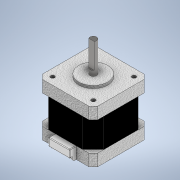
# Autodesk Inventor part: Шаговый двигатель
Saved by Autodesk Inventor 2020 (Build 240168000, 168)
## iProperties
Created: 2020-12-07
Part Number: Шаговый двигатель
Material: Типовые
Document SubType Name: Modeling
Designer: User
Density: 1 g/cm^3
Appearance: По умолчанию
Author: User
Autodesk Inventor part; units mm, degrees
ref_plane "YZ Plane" through (0, 0, 0) normal (1, 0, 0) x (0, 1, 0)
sketch "Эскиз1" plane through (0, 0, 0) normal (0, 1, 0) x (-1, 0, 0)
  line L0 (21.1, 21.1) -> (-21.1, 21.1)
  line L1 (-21.1, 21.1) -> (-21.1, -21.1)
  line L2 (-21.1, -21.1) -> (21.1, -21.1)
  line L3 (21.1, -21.1) -> (21.1, 21.1)
  line L4 (21.1, 21.1) -> (-21.1, -21.1) construction
  line L5 (-21.1, 21.1) -> (21.1, -21.1) construction
  line L6 (-15.5, -15.5) -> (15.5, -15.5) construction
  line L7 (15.5, -15.5) -> (15.5, 15.5) construction
  line L8 (15.5, 15.5) -> (-15.5, 15.5) construction
  line L9 (-15.5, 15.5) -> (-15.5, -15.5) construction
  line L10 (-15.5, -15.5) -> (15.5, 15.5) construction
  line L11 (15.5, -15.5) -> (-15.5, 15.5) construction
  circle A0 centre (15.5, -15.5) radius 1.5
  circle A1 centre (-15.5, -15.5) radius 1.5
  circle A2 centre (15.5, 15.5) radius 1.5
  circle A3 centre (-15.5, 15.5) radius 1.5
  line L12 (21.1, 0) -> (-21.1, 0) construction
  line L13 (0, -21.1) -> (0, 21.1) construction
  point P0 (0, 0)
  dimension "d0" = 42.2
  dimension "d1" = 42.2
  dimension "d2" = 31
  dimension "d3" = 3
  constraints: 28 end point, 8 midpoint, 4 centre point, 4 coincident, 4 parallel, 3 equal radius, 3 perpendicular, 2 horizontal
  measures "d0" distance of L2.end L1.end
  measures "d1" distance of L1.end L0.end
  measures "d2" distance of L8.end L6.start
  measures "d3" diameter of A0
extrude "Выдавливание1" add sketch "Эскиз1" along normal blind 40
sketch "Эскиз2" plane through (0, 40, 0) normal (0, 1, 0) x (1, 0, 0)
  circle A0 centre (0, 0) radius 11
  dimension "d9" = 22
  constraints: 1 centre point, 1 coincident
  measures "d9" diameter of A0
extrude "Выдавливание2" add sketch "Эскиз2" along normal blind 2
sketch "Эскиз3" plane through (0, 42, 0) normal (0, 1, 0) x (1, 0, 0)
  circle A0 centre (0, 0) radius 2.5
  dimension "d12" = 5
  constraints: 1 centre point, 1 coincident
  measures "d12" diameter of A0
extrude "Выдавливание3" add sketch "Эскиз3" along normal blind 23
sketch "Эскиз4" plane through (0, 65, 0) normal (0, 1, 0) x (1, 0, 0)
  circle A0 centre (0, 0) radius 2.5 projected
  line L0 (-2.0766, -1.392) -> (2.0766, -1.392)
  line L1 (-2.4977, 0.108) -> (2.4977, 0.108) construction
  dimension "d15" = 1.5
  constraints: 4 end point, 4 point on circle, 2 horizontal
  measures "d15" distance between parallel lines of L0 L1
extrude "Выдавливание4" cut sketch "Эскиз4" against normal blind 19 contours L0 A0 picked at (0, -1.7613)
ref_plane "РабПлоскость1" through (0, 9, 0) normal (0, -1, 0) x (1, 0, 0)
ref_plane "РабПлоскость2" through (0, 31, 0) normal (0, 1, 0) x (1, 0, 0)
split body "Разделение1" result two bodies by plane through (0, 9, 0) normal (0, -1, 0) first body at (-4.7924, 0.5, 4.8351)
split body "Разделение2" result two bodies by plane through (0, 31, 0) normal (0, 1, 0) bodies 3 first body at (-4.7924, 31.5, -4.8351)
chamfer "Фаска1" distance 3.5 angle 45 8 edges at (-21.1, 4.5, 21.1) (-21.1, 4.5, -21.1) (21.1, 4.5, 21.1) (21.1, 4.5, -21.1) (-21.1, 35.5, -21.1) (-21.1, 35.5, 21.1) (21.1, 35.5, 21.1) (21.1, 35.5, -21.1)
chamfer "Фаска2" distance 8 angle 45 4 edges at (21.1, 20, -21.1) (-21.1, 20, -21.1) (21.1, 20, 21.1) (-21.1, 20, 21.1)
sketch "Эскиз5" plane through (-17.6, 0, 21.1) normal (0, 0, 1) x (1, 0, 0)
  line L0 (25.7, 0) -> (9.5, 0)
  line L1 (9.5, 0) -> (9.5, 9)
  line L2 (9.5, 9) -> (25.7, 9)
  line L3 (25.7, 9) -> (25.7, 0)
  line L4 (0, 0) -> (35.2, 0) projected
  line L5 (0, 9) -> (35.2, 9) projected
  point P0 (17.6, 0)
  point P1 (17.6, 0)
  dimension "d26" = 16.2
  constraints: 8 end point, 2 midpoint, 2 parallel, 1 collinear, 1 horizontal, 1 perpendicular
  measures "d26" distance of L1.end L2.end
extrude "Выдавливание5" add sketch "Эскиз5" along normal blind 5 separate body
sketch "Эскиз6" plane through (-17.6, 0, 26.1) normal (0, 0, 1) x (1, 0, 0)
  line L0 (9.5, 0) -> (25.7, 0)
  line L1 (25.7, 0) -> (25.7, 3)
  line L2 (25.7, 3) -> (9.5, 3)
  line L3 (9.5, 3) -> (9.5, 0)
  line L4 (9.5, 9) -> (9.5, 0) projected
  line L5 (0, 0) -> (35.2, 0) projected
  point P0 (17.6, 0)
  dimension "d30" = 16.2
  dimension "d31" = 3
  constraints: 8 end point, 2 collinear, 2 parallel, 1 horizontal, 1 perpendicular
  measures "d30" distance of L2.end L1.end
  measures "d31" distance of L1.end L0.end
extrude "Выдавливание6" cut sketch "Эскиз6" against normal blind 2 bodies 6
fillet "Сопряжение1" radius 2 1 edges at (0, 0, 24.1)
fillet "Сопряжение1" radius 0.5 8 edges at (8.1, 6, 26.1) (0, 3, 26.1) (-8.1, 6, 26.1) (0, 9, 26.1) (8.1, 9, 23.6) (-8.1, 9, 23.6) (-8.1, 3, 25.1) (8.1, 3, 25.1)
thread "Резьба1" size "M3x0.5" class "6H" standard "ANSI Metric M Profile" full length
thread "Резьба2" size "M3x0.5" class "6H" standard "ANSI Metric M Profile" full length
thread "Резьба3" size "M3x0.5" class "6H" standard "ANSI Metric M Profile" full length
thread "Резьба4" size "M3x0.5" class "6H" standard "ANSI Metric M Profile" full length
equation "\"d1\" = d0"
